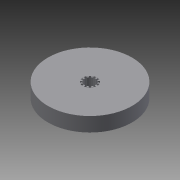
# Autodesk Inventor part: Protector
Saved by Autodesk Inventor 2015 (Build 190159000, 159)
## iProperties
Created: 2015-01-10
Part Number: Protector
Material: Generic
Document SubType Name: Modeling
Designer: harrykuperstein
Density: 1 g/cm^3
Appearance: Default
Author: harrykuperstein
Autodesk Inventor part; units mm, degrees
ref_plane "YZ Plane" through (0, 0, 0) normal (1, 0, 0) x (0, 1, 0)
ref_plane "XZ Plane" through (0, 0, 0) normal (0, 1, 0) x (-1, 0, 0)
ref_plane "XY Plane" through (0, 0, 0) normal (0, 0, 1) x (1, 0, 0)
sketch "Sketch1" plane through (0, 0, 0) normal (0, 1, 0) x (-1, 0, 0)
  circle A0 centre (0, 0) radius 5.2451
  circle A1 centre (0, 0) radius 4.064 construction
  line L0 (4.0236, 0.5715) -> (5.2139, 0.5715)
  line L1 (5.2139, -0.5715) -> (4.0236, -0.5715)
  line L2 (3.7703, 1.5169) -> (4.8011, 2.112)
  line L3 (4.2296, 3.1019) -> (3.1988, 2.5067)
  line L4 (3.1019, 4.2296) -> (2.5067, 3.1988)
  line L5 (2.112, 4.8011) -> (1.5169, 3.7703)
  line L6 (-0.5715, 5.2139) -> (-0.5715, 4.0236)
  line L7 (-2.112, 4.8011) -> (-1.5169, 3.7703)
  line L8 (-3.1019, 4.2296) -> (-2.5067, 3.1988)
  line L9 (-4.8011, 2.112) -> (-3.7703, 1.5169)
  line L10 (-4.2296, 3.1019) -> (-3.1988, 2.5067)
  line L11 (-5.2139, 0.5715) -> (-4.0236, 0.5715)
  line L12 (-5.2139, -0.5715) -> (-4.0236, -0.5715)
  line L13 (-4.8011, -2.112) -> (-3.7703, -1.5169)
  line L14 (-4.2296, -3.1019) -> (-3.1988, -2.5067)
  line L15 (-3.1019, -4.2296) -> (-2.5067, -3.1988)
  line L16 (-2.112, -4.8011) -> (-1.5169, -3.7703)
  line L17 (-0.5715, -5.2139) -> (-0.5715, -4.0236)
  line L18 (0.5715, -5.2139) -> (0.5715, -4.0236)
  line L19 (3.1019, -4.2296) -> (2.5067, -3.1988)
  line L20 (2.112, -4.8011) -> (1.5169, -3.7703)
  line L21 (4.2296, -3.1019) -> (3.1988, -2.5067)
  line L22 (4.8011, -2.112) -> (3.7703, -1.5169)
  line L23 (0.5715, 5.2139) -> (0.5715, 4.0236)
  circle A2 centre (0, 0) radius 30.6451
  circle A3 centre (0, 0) radius 4.064
  line L24 (5.2139, 0.5715) -> (5.2139, -0.5715)
  line L25 (4.0236, 0.5715) -> (4.0236, -0.5715)
  line L26 (3.7703, -1.5169) -> (3.1988, -2.5067)
  line L27 (2.5067, -3.1988) -> (1.5169, -3.7703)
  line L28 (0.5715, -4.0236) -> (-0.5715, -4.0236)
  line L29 (-1.5169, -3.7703) -> (-2.5067, -3.1988)
  line L30 (-3.1988, -2.5067) -> (-3.7703, -1.5169)
  line L31 (-4.0236, -0.5715) -> (-4.0236, 0.5715)
  line L32 (-3.7703, 1.5169) -> (-3.1988, 2.5067)
  line L33 (-2.5067, 3.1988) -> (-1.5169, 3.7703)
  line L34 (-0.5715, 4.0236) -> (0.5715, 4.0236)
  line L35 (1.5169, 3.7703) -> (2.5067, 3.1988)
  line L36 (3.1988, 2.5067) -> (3.7703, 1.5169)
  line L37 (3.7703, 1.5169) -> (4.8011, 2.112)
  line L38 (4.8011, 2.112) -> (4.2296, 3.1019)
  line L39 (3.1019, 4.2296) -> (2.112, 4.8011)
  line L40 (0.5715, 5.2139) -> (-0.5715, 5.2139)
  line L41 (-2.112, 4.8011) -> (-3.1019, 4.2296)
  line L42 (-4.2296, 3.1019) -> (-4.8011, 2.112)
  line L43 (-5.2139, 0.5715) -> (-5.2139, -0.5715)
  line L44 (-3.1019, -4.2296) -> (-2.112, -4.8011)
  line L45 (-4.2296, -3.1019) -> (-4.8011, -2.112)
  line L46 (-0.5715, -5.2139) -> (0.5715, -5.2139)
  line L47 (2.112, -4.8011) -> (3.1019, -4.2296)
  line L48 (4.2296, -3.1019) -> (4.8011, -2.112)
  dimension "d0" = 10.4902
  dimension "d1" = 8.128
  dimension "d4" = 1.143
  dimension "d5" = 1.143
  dimension "d6" = 1.143
  dimension "d7" = 1.143
  dimension "d8" = 1.143
  dimension "d9" = 1.143
  dimension "d11" = 1.143
  dimension "d12" = 30
  dimension "d15" = 30
  dimension "d18" = 30
  dimension "d20" = 1.143
  dimension "d21" = 30
  dimension "d22" = 30
  dimension "d23" = 30
  dimension "d28" = 1.143
  dimension "d29" = 30
  dimension "d30" = 30
  dimension "d31" = 1.143
  dimension "d32" = 30
  dimension "d34" = 1.143
  dimension "d35" = 25.4
  constraints: 98 end point, 19 parallel, 5 perpendicular, 4 coincident, 3 point on line, 2 horizontal, 1 centre point, 1 vertical, 55 other
  measures "d4" distance between parallel lines of L1 L0
  measures "d5" distance between parallel lines of L21 L22
  measures "d6" distance between parallel lines of L3 L2
  measures "d7" distance between parallel lines of L5 L4
  measures "d8" distance between parallel lines of L17 L18
  measures "d9" distance between parallel lines of L13 L14
  measures "d11" distance between parallel lines of L6 L23
  measures "d12" angle of L22 L1
  measures "d15" angle of L16 L17
  measures "d18" angle of L2 L0
  measures "d20" distance between parallel lines of L20 L19
  measures "d21" angle of L19 L21
  measures "d22" angle of L18 L20
  measures "d23" angle of L14 L15
  measures "d28" distance between parallel lines of L11 L12
  measures "d29" angle of L12 L13
  measures "d30" angle of L9 L11
  measures "d31" distance between parallel lines of L8 L7
  measures "d32" angle of L7 L6
  measures "d34" distance between parallel lines of L10 L9
extrude "Extrusion1" add sketch "Sketch1" along normal blind 10.414 contours L24 L1 A3 L0 | L2 A3 L3 L38 | A3 L25 | L48 L21 A3 L22 | L36 A3 | A3 L26 | L4 A3 L5 L39 | L47 L20 A3 L19 | L35 A3 | A3 L27 | L23 A3 L6 L40 | L46 L17 A3 L18 | L34 A3 | A3 L28 | L7 A3 L8 L41 | L44 L15 A3 L16 | L33 A3 | A3 L29 | L10 A3 L9 L42 | L45 L13 A3 L14 | L32 A3 | A3 L30 | L11 A3 L12 L43 | L31 A3 | A2
body "Solid1"
